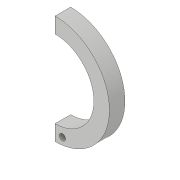
# Autodesk Inventor part: 5
Saved by Autodesk Inventor 2019 (Build 230136000, 136)
## iProperties
Created: 2019-11-17
Part Number: 5
Material: Generic
Document SubType Name: Modeling
Designer: Admin
Density: 1 g/cm^3
Appearance: Default
Author: Admin
Autodesk Inventor part; units mm, degrees
ref_plane "YZ Plane" through (0, 0, 0) normal (1, 0, 0) x (0, 1, 0)
ref_plane "XZ Plane" through (0, 0, 0) normal (0, 1, 0) x (-1, 0, 0)
ref_plane "XY Plane" through (0, 0, 0) normal (0, 0, 1) x (1, 0, 0)
sketch "Sketch1" plane through (0, 0, 0) normal (0, 0, 1) x (1, 0, 0)
  circle A0 centre (0, 0) radius 35
  dimension "d0" = 70
  constraints: 1 centre point, 1 coincident
  measures "d0" diameter of A0
extrude "Extrusion1" add sketch "Sketch1" along normal blind 10
sketch "Sketch2" plane through (0, 0, 10) normal (0, 0, 1) x (1, 0, 0)
  circle A0 centre (0, 0) radius 25
  line L0 (0, 34.925) -> (0, 25)
  line L1 (0, -25) -> (0, -34.925)
  line L2 (0, -30.1625) -> (4.7625, -30.1625)
  circle A1 centre (4.7625, -30.1625) radius 2
  dimension "d3" = 50
  dimension "d4" = 4
  constraints: 6 end point, 3 point on line, 2 centre point, 2 coincident, 2 point on circle, 1 perpendicular, 1 vertical
  measures "d3" diameter of A0
  measures "d4" diameter of A1
extrude "Extrusion2" cut sketch "Sketch2" against normal blind 10
sketch "Sketch3" plane through (0, 0, 10) normal (0, 0, 1) x (1, 0, 0)
  circle A0 centre (0, 0) radius 35 projected
  line L0 (0, 35) -> (0, -35)
  constraints: 2 end point, 2 point on circle, 1 vertical
extrude "Extrusion3" cut sketch "Sketch3" against normal blind 10 contours L0 A0 picked at (-19.0322, -1.7332)
body "Solid1"
